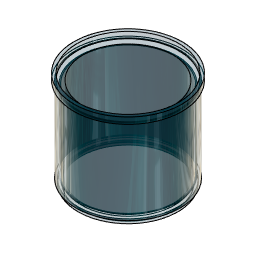
towerlightcylinder v6 (Autodesk Fusion 360 design; units mm, degrees)
Autodesk Fusion 360 part; units mm, degrees
sketch "Sketch1" plane through (0, 0, 0) normal (0, 0, 1) x (1, 0, 0)
  circle A0 centre (0, 0) radius 24.5
  dimension "d1" = 49
  constraint coincident A0.centre origin
  measures "d1" diameter of A0
extrude "Extrude1" add sketch "Sketch1" along normal blind 40 makes body 1
shell "Shell1" thickness 3.5 removed faces 2 at (8.8365, 2.1715, 40) at (8.8365, 2.1715, 0) on bodies 1
sketch "Sketch2" plane through (0, 0, 0) normal (0, 0, 1) x (1, 0, 0)
  circle A0 centre (0, 0) radius 23.5
  dimension "d5" = 47
  constraint coincident A0.centre origin
  measures "d5" diameter of A0
extrude "Extrude2" add sketch "Sketch2" against normal blind 2 bodies 1
shell "Shell2" thickness 1.5 removed faces 2 at (5.7422, 5.328, -2) at (2.2464, 4.4528, 0) on bodies 1
sketch "Sketch3" plane through (0, 0, 0) normal (0, 0, 1) x (1, 0, 0)
ref_plane "WorkPlane1" through (0, 0, 40) normal (0, 0, 1) x (1, 0, 0)
extrude "Extrude3" add 1 faces at (23.1639, -2.2605, 40) along direction (0, 0, 1) blind 2 on bodies 1 bodies 1
split "Split1" by plane through (0, 0, 40) normal (0, 0, 1) bodies 1 makes body 2 at (23.1639, -2.2605, 42)
move_face "OffsetFaces1" offset -2 1 faces at (-20.9739, -1.0468, 41.3333) on bodies 2
copy_body "Body->Comp1" bodies 2 removing the originals makes body 3 in component "Component"
copy_body "Body->Comp2" bodies 1 removing the originals makes body 4 in component "Component'"
move_face "OffsetFaces1'" offset 0.5 1 faces at (-24.3783, 2.4394, 40.6667) on bodies 3 in component "Component"
move_face "OffsetFaces2" offset -0.5 1 faces at (-22.9714, -1.1465, 41.3333) on bodies 3 in component "Component"
move_face "OffsetFaces3" offset 1 1 faces at (24.4069, 1.242, 42) on bodies 3 in component "Component"
move_face "OffsetFaces4" offset 1 1 faces at (-6.771, -24.0656, 41) on bodies 3 in component "Component"
move_face "OffsetFaces5" offset -0.5 1 faces at (-6.3648, -22.6217, 41) on bodies 3 in component "Component"
move_face "OffsetFaces6" offset -0.5 1 faces at (-25.9677, -1.296, 42) on bodies 3 in component "Component"
component "Component" placed x (1, 0, 0) y (0, 1, 0) z (0, 0, 1) at (0, 0, 0)
component "Component'" placed x (1, 0, 0) y (0, 1, 0) z (0, 0, 1) at (0, 0, 0)
